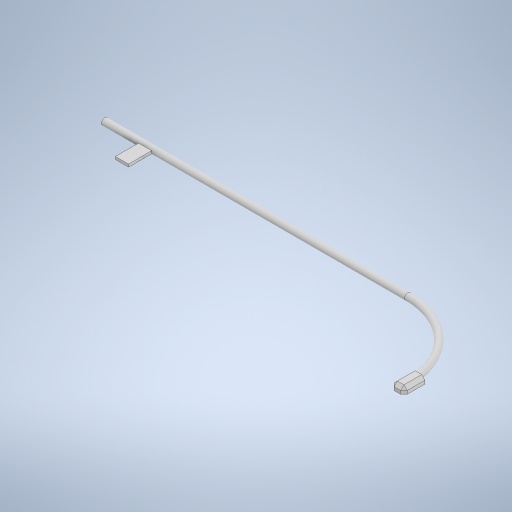
# Autodesk Inventor part: Height adjust(H)
Saved by Autodesk Inventor 2023 (Build 270158030, 158C)
## iProperties
Created: 2023-03-05
Part Number: Height adjust(H)
Material: Generic
Document SubType Name: Modeling
Designer: mpino
Density: 1 g/cm^3
Appearance: Default
Author: mpino
Autodesk Inventor part; units mm, degrees
ref_plane "YZ Plane" through (0, 0, 0) normal (1, 0, 0) x (0, 1, 0)
ref_plane "XZ Plane" through (0, 0, 0) normal (0, 1, 0) x (-1, 0, 0)
ref_plane "XY Plane" through (0, 0, 0) normal (0, 0, 1) x (1, 0, 0)
sketch "Sketch1" plane through (0, 0, 0) normal (1, 0, 0) x (0, 1, 0)
  circle A0 centre (0, 0) radius 3.175
  dimension "d0" = 6.35
  constraints: 1 centre point, 1 coincident
  measures "d0" diameter of A0
sketch "Sketch2" plane through (0, 0, 0) normal (0, 1, 0) x (-1, 0, 0)
  line L0 (0, 0) -> (-292.1, 0)
  arc A0 (-363.942, 71.842) -> (-292.1, 0) centre (-292.1, 71.842) ccw
  line L1 (-292.1, 0) -> (-363.942, 71.842) construction
  line L2 (-292.1, 0) -> (-190.5, 0) construction
  dimension "d1" = 292.1
  dimension "d2" = 101.6
  dimension "d3" = 135
  constraints: 6 end point, 2 horizontal, 2 point on circle, 1 centre point, 1 equal length, 1 tangent
  measures "d1" distance of L0.start L0.end
  measures "d2" distance of L0.end L1.end
  measures "d3" angle of L2 L1
sweep "Sweep1" add profiles "Sketch1" path "Sketch2"
sketch "Sketch3" plane through (0, 0, 0) normal (0, 1, 0) x (-1, 0, 0)
  line L0 (-357.592, 82.002) -> (-370.292, 82.002)
  line L1 (-370.292, 82.002) -> (-370.292, 61.682)
  line L2 (-370.292, 61.682) -> (-357.592, 61.682)
  line L3 (-357.592, 61.682) -> (-357.592, 82.002)
  line L4 (-360.767, 71.842) -> (-367.117, 71.842) projected
  line L5 (-357.592, 82.002) -> (-370.292, 61.682) construction
  line L6 (-370.292, 82.002) -> (-357.592, 61.682) construction
  point P0 (0, 0)
  point P1 (-363.942, 71.842)
  dimension "d6" = 12.7
  dimension "d7" = 20.32
  constraints: 12 end point, 3 midpoint, 2 parallel, 1 horizontal, 1 perpendicular
  measures "d6" distance of L2.end L1.end
  measures "d7" distance of L1.end L0.end
extrude "Extrusion1" add sketch "Sketch3" along normal mid plane 6.35
chamfer "Chamfer1" distance 3.175 angle 45 5 edges at (370.292, 0, 82.002) (357.592, 0, 82.002) (357.592, 3.175, 71.842) (370.292, 3.175, 71.842) (363.942, 3.175, 82.002)
sketch "Sketch4" plane through (0, 0, 0) normal (0, 1, 0) x (-1, 0, 0)
  line L0 (0, 0) -> (-2.54, 0)
  line L1 (-2.54, 0) -> (-81.28, 0)
  line L2 (-35.56, 25.4) -> (-48.26, 25.4)
  line L3 (-48.26, 25.4) -> (-48.26, -25.4)
  line L4 (-48.26, -25.4) -> (-35.56, -25.4)
  line L5 (-35.56, -25.4) -> (-35.56, 25.4)
  line L6 (-35.56, 25.4) -> (-48.26, -25.4) construction
  line L7 (-48.26, 25.4) -> (-35.56, -25.4) construction
  line L8 (-35.56, 0) -> (-48.26, 0)
  point P0 (-41.91, 0)
  point P1 (-48.26, 0)
  point P2 (-35.56, 0)
  dimension "d13" = 2.54
  dimension "d14" = 78.74
  dimension "d15" = 12.7
  dimension "d16" = 50.8
  constraints: 18 end point, 5 midpoint, 2 horizontal, 2 parallel, 1 perpendicular, 1 point on line
  measures "d13" distance of L0.start L0.end
  measures "d14" distance of L0.end L1.end
  measures "d15" distance of L4.end L3.end
  measures "d16" distance between parallel lines of L2 L4
extrude "Extrusion2" add sketch "Sketch4" along normal mid plane 2.54 contours L1 L3 L2 L5
body "Solid1"
